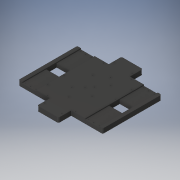
# Autodesk Inventor part: BottomPlateV2
Saved by Autodesk Inventor 2017 (Build 210142000, 142)
## iProperties
Created: 2017-03-10
Part Number: BottomPlateV2
Material: Polyethylene, High Density
Document SubType Name: Modeling
Designer: Naga
Density: 0.952 g/cm^3
Appearance: Smooth - Black
Author: Naga
Autodesk Inventor part; units mm, degrees
ref_plane "YZ Plane" through (0, 0, 0) normal (1, 0, 0) x (0, 1, 0)
ref_plane "XZ Plane" through (0, 0, 0) normal (0, 1, 0) x (-1, 0, 0)
ref_plane "XY Plane" through (0, 0, 0) normal (0, 0, 1) x (1, 0, 0)
sketch "Sketch1" plane through (0, 0, 0) normal (0, 1, 0) x (-1, 0, 0)
  line L0 (0, 0) -> (228.6, 0)
  line L1 (228.6, 0) -> (228.6, -228.6)
  line L2 (228.6, -228.6) -> (0, -228.6)
  line L3 (0, -228.6) -> (0, 0)
  line L4 (0, 0) -> (59.9999, 0)
  line L5 (59.9999, 0) -> (59.9999, -28.3972)
  line L6 (59.9999, -28.3972) -> (0, -28.3972)
  line L7 (0, -28.3972) -> (0, 0)
  line L8 (114.3, 0) -> (114.3, -114.3) construction
  line L9 (114.3, -114.3) -> (0, -114.3) construction
  line L10 (228.6, 0) -> (0, 0)
  line L11 (228.6, -228.6) -> (228.6, 0)
  line L12 (228.6, 0) -> (168.6001, 0)
  line L13 (168.6001, 0) -> (168.6001, -28.3972)
  line L14 (168.6001, -28.3972) -> (228.6, -28.3972)
  line L15 (228.6, -28.3972) -> (228.6, 0)
  line L16 (228.6, -228.6) -> (228.6, 0)
  line L17 (0, 0) -> (0, -228.6)
  line L18 (0, -228.6) -> (59.9999, -228.6)
  line L19 (59.9999, -228.6) -> (59.9999, -200.2028)
  line L20 (59.9999, -200.2028) -> (0, -200.2028)
  line L21 (0, -200.2028) -> (0, -228.6)
  line L22 (228.6, 0) -> (228.6, -228.6)
  line L23 (228.6, -228.6) -> (168.6001, -228.6)
  line L24 (168.6001, -228.6) -> (168.6001, -200.2028)
  line L25 (168.6001, -200.2028) -> (228.6, -200.2028)
  line L26 (228.6, -200.2028) -> (228.6, -228.6)
  dimension "d0" = 228.6
  dimension "d1" = 228.6
  dimension "d2" = 59.9999
  dimension "d3" = 28.3972
  constraints: 54 end point, 17 symmetric about line, 4 parallel, 2 horizontal, 2 midpoint, 2 perpendicular, 1 vertical
  measures "d0" distance of L1.end L2.end
  measures "d1" distance of L0.end L1.end
  measures "d2" distance of L5.end L6.end
  measures "d3" distance of L4.end L5.end
extrude "Extrusion1" add sketch "Sketch1" along normal blind 12.7 contours L0 L13 L14 L1 L25 L24 L2 L19 L20 L3 L6 L5
sketch "Sketch2" plane through (0, 12.7, 0) normal (0, 1, 0) x (1, 0, 0)
  line L0 (-59.9999, 200.2028) -> (-59.9999, 228.6) projected
  line L1 (-59.9999, 228.6) -> (-168.6001, 228.6) projected
  line L2 (-168.6001, 228.6) -> (-168.6001, 200.2028) projected
  line L3 (-168.6001, 200.2028) -> (-228.6, 200.2028) projected
  line L4 (-228.6, 200.2028) -> (-228.6, 28.3972) projected
  line L5 (-228.6, 28.3972) -> (-168.6001, 28.3972) projected
  line L6 (-168.6001, 28.3972) -> (-168.6001, 0) projected
  line L7 (-168.6001, 0) -> (-59.9999, 0) projected
  line L8 (-59.9999, 0) -> (-59.9999, 28.3972) projected
  line L9 (-59.9999, 28.3972) -> (0, 28.3972) projected
  line L10 (0, 28.3972) -> (0, 200.2028) projected
  line L11 (0, 200.2028) -> (-59.9999, 200.2028) projected
  line L12 (-228.6, 28.3972) -> (-168.6001, 28.3972) projected
  line L13 (-198.6001, 28.3972) -> (-198.6001, 34.7472) construction
  line L14 (-228.6, 200.2028) -> (-228.6, 28.3972) projected
  line L15 (-228.6, 34.7472) -> (-219.075, 34.7472) construction
  line L16 (-228.6, 34.7472) -> (-219.075, 34.7472) construction
  line L17 (-219.075, 34.7472) -> (-180.975, 34.7472)
  line L18 (-180.975, 34.7472) -> (-180.975, 44.2722)
  line L19 (-180.975, 44.2722) -> (-219.075, 44.2722)
  line L20 (-219.075, 44.2722) -> (-219.075, 34.7472)
  line L21 (-200.025, 44.2722) -> (-200.025, 39.5097) construction
  line L22 (-200.025, 39.5097) -> (-219.075, 39.5097) construction
  circle A0 centre (-200.025, 39.5097) radius 1.5875
  line L23 (-200.025, 39.5097) -> (-214.825, 39.5097)
  circle A1 centre (-214.825, 39.5097) radius 1.5875
  circle A2 centre (-185.225, 39.5097) radius 1.5875
  line L24 (-228.6, 200.2028) -> (-228.6, 28.3972) projected
  line L25 (-228.6, 114.3) -> (-114.3, 114.3) construction
  line L26 (-114.3, 114.3) -> (-114.3, 0) construction
  line L27 (-29.9999, 28.3972) -> (-29.9999, 34.7472) construction
  line L28 (0, 34.7472) -> (-9.525, 34.7472) construction
  line L29 (0, 34.7472) -> (-9.525, 34.7472) construction
  line L30 (-9.525, 34.7472) -> (-47.625, 34.7472)
  line L31 (-47.625, 34.7472) -> (-47.625, 44.2722)
  line L32 (-47.625, 44.2722) -> (-9.525, 44.2722)
  line L33 (-9.525, 44.2722) -> (-9.525, 34.7472)
  line L34 (-28.575, 44.2722) -> (-28.575, 39.5097) construction
  line L35 (-28.575, 39.5097) -> (-9.525, 39.5097) construction
  circle A3 centre (-28.575, 39.5097) radius 1.5875
  line L36 (-28.575, 39.5097) -> (-13.775, 39.5097)
  circle A4 centre (-13.775, 39.5097) radius 1.5875
  circle A5 centre (-43.375, 39.5097) radius 1.5875
  line L37 (-198.6001, 200.2028) -> (-198.6001, 193.8528) construction
  line L38 (-228.6, 193.8528) -> (-219.075, 193.8528) construction
  line L39 (-228.6, 193.8528) -> (-219.075, 193.8528) construction
  line L40 (-219.075, 193.8528) -> (-180.975, 193.8528)
  line L41 (-180.975, 193.8528) -> (-180.975, 184.3278)
  line L42 (-180.975, 184.3278) -> (-219.075, 184.3278)
  line L43 (-219.075, 184.3278) -> (-219.075, 193.8528)
  line L44 (-200.025, 184.3278) -> (-200.025, 189.0903) construction
  line L45 (-200.025, 189.0903) -> (-219.075, 189.0903) construction
  circle A6 centre (-200.025, 189.0903) radius 1.5875
  line L46 (-200.025, 189.0903) -> (-214.825, 189.0903)
  circle A7 centre (-214.825, 189.0903) radius 1.5875
  circle A8 centre (-185.225, 189.0903) radius 1.5875
  line L47 (-114.3, 114.3) -> (-114.3, 228.6) construction
  line L48 (-47.625, 193.8528) -> (-47.625, 184.3278)
  circle A9 centre (-43.375, 189.0903) radius 1.5875
  circle A10 centre (-28.575, 189.0903) radius 1.5875
  line L49 (-29.9999, 200.2028) -> (-29.9999, 193.8528) construction
  line L50 (-47.625, 184.3278) -> (-9.525, 184.3278)
  line L51 (-9.525, 184.3278) -> (-9.525, 193.8528)
  line L52 (0, 193.8528) -> (-9.525, 193.8528) construction
  line L53 (0, 193.8528) -> (-9.525, 193.8528) construction
  line L54 (-9.525, 193.8528) -> (-47.625, 193.8528)
  line L55 (-28.575, 189.0903) -> (-13.775, 189.0903)
  line L56 (-28.575, 189.0903) -> (-9.525, 189.0903) construction
  circle A11 centre (-13.775, 189.0903) radius 1.5875
  line L57 (-28.575, 184.3278) -> (-28.575, 189.0903) construction
  point P0 (0, 0)
  dimension "d6" = 6.35
  dimension "d7" = 9.525
  dimension "d8" = 0
  dimension "d9" = 38.1
  dimension "d10" = 9.525
  dimension "d11" = 3.175
  dimension "d12" = 14.8
  dimension "d13" = 3.175
  constraints: 86 end point, 47 symmetric about line, 12 centre point, 8 coincident, 5 midpoint, 5 point on line, 3 horizontal, 3 perpendicular, 2 parallel, 2 vertical, 1 collinear, 10 other
  measures "d6" distance of L13.start L13.end
  measures "d7" distance of L15.start L15.end
  measures "d8" distance between parallel lines of L15 L16
  measures "d9" distance of L19.end L18.end
  measures "d10" distance of L18.end L17.end
  measures "d11" diameter of A0
  measures "d12" distance of L23.start L23.end
  measures "d13" diameter of A1
extrude "Extrusion2" cut sketch "Sketch2" against normal blind 0.7937 contours L20 L19 L18 L17 | L30 L31 L32 L33 | L40 L41 L42 L43 | L54 L51 L50 L48
sketch "Sketch3" plane through (0, 0, 0) normal (0, -1, 0) x (1, 0, 0)
  circle A0 centre (-13.775, -39.5097) radius 1.5875 projected
  circle A1 centre (-28.575, -39.5097) radius 1.5875 projected
  circle A2 centre (-43.375, -39.5097) radius 1.5875 projected
  circle A3 centre (-13.775, -189.0903) radius 1.5875 projected
  circle A4 centre (-28.575, -189.0903) radius 1.5875 projected
  circle A5 centre (-43.375, -189.0903) radius 1.5875 projected
  circle A6 centre (-185.225, -189.0903) radius 1.5875 projected
  circle A7 centre (-200.025, -189.0903) radius 1.5875 projected
  circle A8 centre (-214.825, -189.0903) radius 1.5875 projected
  circle A9 centre (-214.825, -39.5097) radius 1.5875 projected
  circle A10 centre (-200.025, -39.5097) radius 1.5875 projected
  circle A11 centre (-185.225, -39.5097) radius 1.5875 projected
  point P0 (0, 0)
extrude "Extrusion3" cut sketch "Sketch3" against normal up to surface (12.7 mm away)
sketch "Sketch4" plane through (0, 12.7, 0) normal (0, 1, 0) x (1, 0, 0)
  line L0 (-219.075, 184.3278) -> (-219.075, 193.8528) projected
  line L1 (-219.075, 193.8528) -> (-180.975, 193.8528)
  line L2 (-180.975, 193.8528) -> (-180.975, 34.7472)
  line L3 (-180.975, 34.7472) -> (-219.075, 34.7472)
  line L4 (-219.075, 34.7472) -> (-219.075, 193.8528)
  line L5 (-47.625, 193.8528) -> (-9.525, 193.8528) projected
  line L6 (-9.525, 44.2722) -> (-9.525, 34.7472) projected
  line L7 (-47.625, 193.8528) -> (-9.525, 193.8528)
  line L8 (-9.525, 193.8528) -> (-9.525, 34.7472)
  line L9 (-9.525, 34.7472) -> (-47.625, 34.7472)
  line L10 (-47.625, 34.7472) -> (-47.625, 193.8528)
  point P0 (0, 0)
  constraints: 16 end point, 4 parallel, 2 horizontal, 2 perpendicular
extrude "Extrusion4" cut sketch "Sketch4" against normal blind 3.175
sketch "Sketch5" plane through (0, 12.7, 0) normal (0, 1, 0) x (1, 0, 0)
  line L0 (-168.6001, 0) -> (-59.9999, 0) projected
  line L1 (-114.3, 0) -> (-114.3, 38.1)
  line L2 (-228.6, 200.2028) -> (-228.6, 28.3972) projected
  line L3 (-228.6, 38.1) -> (-152.4, 38.1)
  circle A0 centre (-152.4, 38.1) radius 1.5875
  line L4 (-228.6, 114.3) -> (-127.0378, 114.3)
  circle A1 centre (-76.2, 38.1) radius 1.5875
  circle A2 centre (-152.4, 190.5) radius 1.5875
  circle A3 centre (-76.2, 190.5) radius 1.5875
  point P0 (0, 0)
  dimension "d20" = 38.1
  dimension "d21" = 76.2
  dimension "d22" = 3.175
  constraints: 6 end point, 4 centre point, 4 symmetric about line, 2 coincident, 2 horizontal, 2 midpoint, 1 parallel, 1 point on line, 3 other
  measures "d20" distance of L1.start L1.end
  measures "d21" distance of L3.start L3.end
  measures "d22" diameter of A0
extrude "Extrusion5" cut sketch "Sketch5" against normal up to surface (12.7 mm away)
sketch "Sketch7" plane through (0, 12.7, 0) normal (0, 1, 0) x (1, 0, 0)
  circle A0 centre (-152.4, 190.5) radius 1.5875 projected
  circle A1 centre (-76.2, 190.5) radius 1.5875 projected
  circle A2 centre (-76.2, 38.1) radius 1.5875 projected
  circle A3 centre (-152.4, 38.1) radius 1.5875 projected
  line L0 (-59.9999, 200.2028) -> (-59.9999, 228.6) projected
  line L1 (-59.9999, 228.6) -> (-168.6001, 228.6) projected
  line L2 (-168.6001, 228.6) -> (-168.6001, 200.2028) projected
  line L3 (-168.6001, 200.2028) -> (-228.6, 200.2028) projected
  line L4 (-228.6, 200.2028) -> (-228.6, 28.3972) projected
  line L5 (-228.6, 28.3972) -> (-168.6001, 28.3972) projected
  line L6 (-168.6001, 28.3972) -> (-168.6001, 0) projected
  line L7 (-168.6001, 0) -> (-59.9999, 0) projected
  line L8 (-59.9999, 0) -> (-59.9999, 28.3972) projected
  line L9 (-59.9999, 28.3972) -> (0, 28.3972) projected
  line L10 (0, 28.3972) -> (0, 200.2028) projected
  line L11 (0, 200.2028) -> (-59.9999, 200.2028) projected
  line L12 (-47.625, 34.7472) -> (-47.625, 193.8528) projected
  line L13 (-47.625, 193.8528) -> (-9.525, 193.8528) projected
  line L14 (-9.525, 193.8528) -> (-9.525, 34.7472) projected
  line L15 (-9.525, 34.7472) -> (-47.625, 34.7472) projected
  line L16 (-219.075, 34.7472) -> (-219.075, 193.8528) projected
  line L17 (-219.075, 193.8528) -> (-180.975, 193.8528) projected
  line L18 (-180.975, 193.8528) -> (-180.975, 34.7472) projected
  line L19 (-180.975, 34.7472) -> (-219.075, 34.7472) projected
  line L20 (-228.6, 228.6) -> (-142.875, 228.6)
  line L21 (-228.6, 200.2028) -> (-228.6, 228.6)
  line L22 (0, 228.6) -> (-85.725, 228.6)
  line L23 (0, 200.2028) -> (0, 228.6)
  line L24 (0, 0) -> (-85.725, 0)
  line L25 (-85.725, 0) -> (-85.725, 34.7472)
  line L26 (-85.725, 34.7472) -> (0, 34.7472)
  line L27 (0, 34.7472) -> (0, 0)
  line L28 (-228.6, 0) -> (-142.875, 0)
  line L29 (-142.875, 0) -> (-142.875, 34.7472)
  line L30 (-142.875, 34.7472) -> (-228.6, 34.7472)
  line L31 (-228.6, 34.7472) -> (-228.6, 0)
  line L32 (-228.6, 228.6) -> (-142.875, 228.6)
  line L33 (-142.875, 228.6) -> (-142.875, 193.8528)
  line L34 (-142.875, 193.8528) -> (-228.6, 193.8528)
  line L35 (-228.6, 193.8528) -> (-228.6, 228.6)
  line L36 (0, 28.3972) -> (0, 200.2028) projected
  line L37 (0, 193.8528) -> (-85.725, 193.8528)
  line L38 (-85.725, 193.8528) -> (-85.725, 228.6)
  line L39 (-85.725, 228.6) -> (0, 228.6)
  line L40 (0, 228.6) -> (0, 193.8528)
  dimension "d30" = 34.7472
  constraints: 40 end point, 8 parallel, 6 horizontal, 4 perpendicular, 4 point on line
  measures "d30" distance of L24.end L25.end
extrude "Extrusion7" cut sketch "Sketch7" against normal blind 25.4 contours L11 L10 L37 L13 L38 L1 L0 | L0 L22 L23 L11 | L33 L34 L17 L4 L3 L2 L1 | L10 L9 L8 L7 L25 L26 L15 | L2 L3 L21 L20 | L27 L24 L8 L9 | L30 L29 L7 L6 L5 L4 L19 | L5 L6 L28 L31
sketch "Sketch8" plane through (0, 12.7, 0) normal (0, 1, 0) x (1, 0, 0)
  circle A0 centre (-214.825, 189.0903) radius 1.5875 projected
  circle A1 centre (-185.225, 189.0903) radius 1.5875 projected
  circle A2 centre (-28.575, 189.0903) radius 1.5875 projected
  circle A3 centre (-43.375, 39.5097) radius 1.5875 projected
  circle A4 centre (-13.775, 39.5097) radius 1.5875 projected
  circle A5 centre (-28.575, 39.5097) radius 1.5875 projected
  circle A6 centre (-13.775, 189.0903) radius 1.5875 projected
  circle A7 centre (-43.375, 189.0903) radius 1.5875 projected
  circle A8 centre (-200.025, 189.0903) radius 1.5875 projected
  circle A9 centre (-214.825, 39.5097) radius 1.5875 projected
  circle A10 centre (-185.225, 39.5097) radius 1.5875 projected
  circle A11 centre (-200.025, 39.5097) radius 1.5875 projected
  circle A12 centre (-152.4, 38.1) radius 1.5875 projected
  circle A13 centre (-76.2, 38.1) radius 1.5875 projected
  circle A14 centre (-76.2, 190.5) radius 1.5875 projected
  circle A15 centre (-152.4, 190.5) radius 1.5875 projected
  line L0 (-142.875, 0) -> (-142.875, 34.7472) projected
  line L1 (-142.875, 34.7472) -> (-228.6, 34.7472) projected
  line L2 (-228.6, 193.8528) -> (-228.6, 34.7472) projected
  line L3 (-228.6, 193.8528) -> (-142.875, 193.8528) projected
  line L4 (-142.875, 193.8528) -> (-142.875, 228.6) projected
  line L5 (-85.725, 228.6) -> (-142.875, 228.6) projected
  line L6 (-85.725, 228.6) -> (-85.725, 193.8528) projected
  line L7 (-85.725, 193.8528) -> (0, 193.8528) projected
  line L8 (0, 34.7472) -> (0, 193.8528) projected
  line L9 (0, 34.7472) -> (-85.725, 34.7472) projected
  line L10 (-85.725, 34.7472) -> (-85.725, 0) projected
  line L11 (-142.875, 0) -> (-85.725, 0) projected
  line L12 (-142.875, 0) -> (-85.725, 0) projected
  line L13 (-142.875, 0) -> (-138.5062, 0)
  line L14 (-138.5062, 0) -> (-138.5062, 89.9922)
  line L15 (-138.5062, 89.9922) -> (-142.875, 89.9922)
  line L16 (-142.875, 89.9922) -> (-142.875, 0)
  line L17 (-142.875, 0) -> (-142.875, 34.7472) projected
  line L18 (-138.5062, 0) -> (-142.875, 0)
  line L19 (-142.875, 0) -> (-142.875, 16.002)
  line L20 (-142.875, 16.002) -> (-138.5062, 16.002)
  line L21 (-138.5062, 16.002) -> (-138.5062, 0)
  line L22 (-85.725, 0) -> (-90.0938, 0)
  line L23 (-90.0938, 0) -> (-90.0938, 14.5034)
  line L24 (-90.0938, 14.5034) -> (-85.725, 14.5034)
  line L25 (-85.725, 14.5034) -> (-85.725, 0)
  line L26 (-85.725, 0) -> (-90.0938, 0)
  line L27 (-90.0938, 0) -> (-90.0938, 96.4946)
  line L28 (-90.0938, 96.4946) -> (-85.725, 96.4946)
  line L29 (-85.725, 96.4946) -> (-85.725, 0)
  circle A16 centre (-138.5062, 89.9922) radius 1.5875
  circle A17 centre (-90.0938, 96.4946) radius 1.5875
  circle A18 centre (-90.0938, 14.5034) radius 1.5875
  circle A19 centre (-138.5062, 16.002) radius 1.5875
  point P0 (0, 0)
  dimension "d33" = 4.3688
  dimension "d34" = 89.9922
  dimension "d35" = 16.002
  dimension "d36" = 4.3688
  dimension "d37" = 14.5034
  dimension "d38" = 96.4946
  dimension "d39" = 3.175
  dimension "d40" = 3.175
  dimension "d41" = 3.175
  dimension "d42" = 3.175
  dimension "d74" = 4.3688
  constraints: 32 end point, 8 parallel, 4 centre point, 4 coincident, 4 horizontal, 4 perpendicular, 1 point on line
  measures "d33" distance of L15.end L14.end
  measures "d34" distance of L14.end L13.end
  measures "d35" distance of L18.end L19.end
  measures "d36" distance of L23.end L24.end
  measures "d37" distance of L22.end L23.end
  measures "d38" distance of L26.end L27.end
  measures "d39" diameter of A16
  measures "d40" diameter of A17
  measures "d41" diameter of A18
  measures "d42" diameter of A19
  measures "d74" distance of L27.end L28.end
extrude "ardMount" cut sketch "Sketch8" against normal up to surface (12.7 mm away) contours A19 L14 L20 | L20 L14 A19 | L14 A19 | A18 L27 L23 | L23 L24 A18 | A16 L14 L15 | L15 L14 A16 | L27 A18 L24 | A17 L28 L27 | L27 L28 A17
sketch "Sketch9" plane through (0, 12.7, 0) normal (0, 1, 0) x (1, 0, 0)
  circle A0 centre (-138.5062, 16.002) radius 1.5875 projected
  circle A1 centre (-90.0938, 14.5034) radius 1.5875 projected
  circle A2 centre (-138.5062, 89.9922) radius 1.5875 projected
  circle A3 centre (-90.0938, 96.4946) radius 1.5875 projected
  line L0 (-142.875, 34.7472) -> (-142.875, 0) projected
  line L1 (-142.875, 0) -> (-85.725, 0) projected
  line L2 (-85.725, 0) -> (-85.725, 34.7472) projected
  line L3 (-85.725, 34.7472) -> (-47.625, 34.7472) projected
  line L4 (-47.625, 34.7472) -> (-47.625, 193.8528) projected
  line L5 (-47.625, 193.8528) -> (-85.725, 193.8528) projected
  line L6 (-85.725, 193.8528) -> (-85.725, 228.6) projected
  line L7 (-85.725, 228.6) -> (-142.875, 228.6) projected
  line L8 (-142.875, 228.6) -> (-142.875, 193.8528) projected
  line L9 (-142.875, 193.8528) -> (-180.975, 193.8528) projected
  line L10 (-180.975, 193.8528) -> (-180.975, 34.7472) projected
  line L11 (-180.975, 34.7472) -> (-142.875, 34.7472) projected
  circle A4 centre (-152.4, 190.5) radius 1.5875 projected
  circle A5 centre (-76.2, 190.5) radius 1.5875 projected
  circle A6 centre (-76.2, 38.1) radius 1.5875 projected
  circle A7 centre (-152.4, 38.1) radius 1.5875 projected
  line L12 (-85.725, 228.6) -> (-142.875, 228.6) projected
  line L13 (-114.3, 228.6) -> (-114.3, 148.6607) construction
  line L14 (-142.875, 228.6) -> (-138.7856, 228.6) construction
  line L15 (-138.7856, 228.6) -> (-138.7856, 204.978) construction
  line L16 (-138.7856, 204.978) -> (-142.875, 204.978) construction
  line L17 (-142.875, 204.978) -> (-142.875, 228.6) construction
  line L18 (-142.875, 228.6) -> (-142.875, 193.8528) construction
  line L19 (-142.875, 228.6) -> (-138.7856, 228.6) construction
  line L20 (-138.7856, 228.6) -> (-138.7856, 147.066) construction
  line L21 (-138.7856, 147.066) -> (-142.875, 147.066) construction
  line L22 (-142.875, 147.066) -> (-142.875, 228.6) construction
  circle A8 centre (-138.7856, 204.978) radius 1.5875
  circle A9 centre (-138.7856, 147.066) radius 1.5875
  circle A10 centre (-89.8144, 204.978) radius 1.5875
  circle A11 centre (-89.8144, 147.066) radius 1.5875
  point P0 (0, 0)
  dimension "d45" = 4.0894
  dimension "d46" = 23.622
  dimension "d47" = 81.534
  dimension "d48" = 3.175
  dimension "d49" = 3.175
  constraints: 18 end point, 4 centre point, 4 parallel, 2 coincident, 2 horizontal, 2 perpendicular, 2 symmetric about line, 1 midpoint, 1 point on line, 1 vertical, 2 other
  measures "d45" distance of L15.end L16.end
  measures "d46" distance of L14.end L15.end
  measures "d47" distance of L19.end L20.end
  measures "d48" diameter of A8
  measures "d49" diameter of A9
extrude "piMount" cut sketch "Sketch9" against normal up to surface (12.7 mm away) contours A8 | A9 | A10 | A11
sketch "Sketch10" plane through (0, 0, 0) normal (0, -1, 0) x (1, 0, 0)
  circle A0 centre (-89.8144, -204.978) radius 1.5875 projected
  circle A1 centre (-89.8144, -147.066) radius 1.5875 projected
  circle A2 centre (-138.7856, -147.066) radius 1.5875 projected
  circle A3 centre (-138.7856, -204.978) radius 1.5875 projected
  circle A4 centre (-138.5062, -16.002) radius 1.5875 projected
  circle A5 centre (-90.0938, -14.5034) radius 1.5875 projected
  circle A6 centre (-138.5062, -89.9922) radius 1.5875 projected
  circle A7 centre (-90.0938, -96.4946) radius 1.5875 projected
  circle A8 centre (-214.825, -189.0903) radius 1.5875 projected
  circle A9 centre (-185.225, -189.0903) radius 1.5875 projected
  circle A10 centre (-28.575, -189.0903) radius 1.5875 projected
  circle A11 centre (-43.375, -39.5097) radius 1.5875 projected
  circle A12 centre (-13.775, -39.5097) radius 1.5875 projected
  circle A13 centre (-28.575, -39.5097) radius 1.5875 projected
  circle A14 centre (-13.775, -189.0903) radius 1.5875 projected
  circle A15 centre (-43.375, -189.0903) radius 1.5875 projected
  circle A16 centre (-200.025, -189.0903) radius 1.5875 projected
  circle A17 centre (-214.825, -39.5097) radius 1.5875 projected
  circle A18 centre (-185.225, -39.5097) radius 1.5875 projected
  circle A19 centre (-200.025, -39.5097) radius 1.5875 projected
  circle A20 centre (-152.4, -38.1) radius 1.5875 projected
  circle A21 centre (-76.2, -38.1) radius 1.5875 projected
  circle A22 centre (-76.2, -190.5) radius 1.5875 projected
  circle A23 centre (-152.4, -190.5) radius 1.5875 projected
  line L0 (-142.875, 0) -> (-142.875, -34.7472) projected
  line L1 (-142.875, -34.7472) -> (-228.6, -34.7472) projected
  line L2 (-228.6, -193.8528) -> (-228.6, -34.7472) projected
  line L3 (-228.6, -193.8528) -> (-142.875, -193.8528) projected
  line L4 (-142.875, -193.8528) -> (-142.875, -228.6) projected
  line L5 (-85.725, -228.6) -> (-142.875, -228.6) projected
  line L6 (-85.725, -228.6) -> (-85.725, -193.8528) projected
  line L7 (-85.725, -193.8528) -> (0, -193.8528) projected
  line L8 (0, -34.7472) -> (0, -193.8528) projected
  line L9 (0, -34.7472) -> (-85.725, -34.7472) projected
  line L10 (-85.725, -34.7472) -> (-85.725, 0) projected
  line L11 (-142.875, 0) -> (-85.725, 0) projected
  line L12 (-142.875, -34.7472) -> (-228.6, -34.7472) construction
  line L13 (-228.6, -34.7472) -> (-177.1396, -34.7472) construction
  line L14 (-177.1396, -34.7472) -> (-177.1396, -107.3912) construction
  line L15 (-177.1396, -107.3912) -> (-228.6, -107.3912) construction
  line L16 (-228.6, -107.3912) -> (-228.6, -34.7472) construction
  line L17 (-228.6, -34.7472) -> (-177.1396, -34.7472) construction
  line L18 (-177.1396, -34.7472) -> (-177.1396, -63.1952) construction
  line L19 (-177.1396, -63.1952) -> (-228.6, -63.1952) construction
  line L20 (-228.6, -63.1952) -> (-228.6, -34.7472) construction
  line L21 (-228.6, -34.7472) -> (-120.015, -34.7472) construction
  line L22 (-120.015, -34.7472) -> (-120.015, -107.3912) construction
  line L23 (-120.015, -107.3912) -> (-228.6, -107.3912) construction
  line L24 (-228.6, -107.3912) -> (-228.6, -34.7472) construction
  line L25 (-228.6, -34.7472) -> (-120.015, -34.7472) construction
  line L26 (-120.015, -34.7472) -> (-120.015, -63.1952) construction
  line L27 (-120.015, -63.1952) -> (-228.6, -63.1952) construction
  line L28 (-228.6, -63.1952) -> (-228.6, -34.7472) construction
  line L29 (-85.725, -193.8528) -> (0, -193.8528) construction
  line L30 (0, -193.8528) -> (-51.4604, -193.8528) construction
  line L31 (-51.4604, -193.8528) -> (-51.4604, -121.2088) construction
  line L32 (-51.4604, -121.2088) -> (0, -121.2088) construction
  line L33 (0, -121.2088) -> (0, -193.8528) construction
  line L34 (0, -34.7472) -> (0, -193.8528) construction
  line L35 (0, -193.8528) -> (-51.4604, -193.8528) construction
  line L36 (-51.4604, -193.8528) -> (-51.4604, -165.4048) construction
  line L37 (-51.4604, -165.4048) -> (0, -165.4048) construction
  line L38 (0, -165.4048) -> (0, -193.8528) construction
  line L39 (0, -193.8528) -> (-108.585, -193.8528) construction
  line L40 (-108.585, -193.8528) -> (-108.585, -121.2342) construction
  line L41 (-108.585, -121.2342) -> (0, -121.2342) construction
  line L42 (0, -121.2342) -> (0, -193.8528) construction
  line L43 (0, -193.8528) -> (-108.585, -193.8528) construction
  line L44 (-108.585, -193.8528) -> (-108.585, -165.4048) construction
  line L45 (-108.585, -165.4048) -> (0, -165.4048) construction
  line L46 (0, -165.4048) -> (0, -193.8528) construction
  circle A24 centre (-108.585, -121.2342) radius 1.5875
  circle A25 centre (-108.585, -165.4048) radius 1.5875
  circle A26 centre (-51.4604, -165.4048) radius 1.5875
  circle A27 centre (-51.4604, -121.2088) radius 1.5875
  circle A28 centre (-177.1396, -107.3912) radius 1.5875
  circle A29 centre (-177.1396, -63.1952) radius 1.5875
  circle A30 centre (-120.015, -63.1952) radius 1.5875
  circle A31 centre (-120.015, -107.3912) radius 1.5875
  point P0 (0, 0)
  dimension "d52" = 51.4604
  dimension "d53" = 72.644
  dimension "d54" = 28.448
  dimension "d55" = 108.585
  dimension "d56" = 51.4604
  dimension "d57" = 72.644
  dimension "d58" = 28.448
  dimension "d59" = 108.585
  dimension "d60" = 3.175
  dimension "d61" = 3.175
  dimension "d62" = 3.175
  dimension "d63" = 3.175
  dimension "d64" = 3.175
  dimension "d65" = 3.175
  dimension "d66" = 3.175
  dimension "d67" = 3.175
  constraints: 64 end point, 16 parallel, 8 centre point, 8 coincident, 8 horizontal, 8 perpendicular, 7 point on line
  measures "d52" distance of L14.end L15.end
  measures "d53" distance of L13.end L14.end
  measures "d54" distance of L17.end L18.end
  measures "d55" distance of L22.end L23.end
  measures "d56" distance of L31.end L32.end
  measures "d57" distance of L30.end L31.end
  measures "d58" distance of L35.end L36.end
  measures "d59" distance of L40.end L41.end
  measures "d60" diameter of A24
  measures "d61" diameter of A25
  measures "d62" diameter of A26
  measures "d63" diameter of A27
  measures "d64" diameter of A28
  measures "d65" diameter of A29
  measures "d66" diameter of A30
  measures "d67" diameter of A31
extrude "sabertoothMount" cut sketch "Sketch10" against normal up to surface (12.7 mm away) contours A24 | A25 | A26 | A27 | A28 | A29 | A30 | A31
sketch "Sketch11" plane through (0, 0, 0) normal (0, -1, 0) x (1, 0, 0)
  line L0 (-47.625, -34.7472) -> (-47.625, -193.8528) projected
  circle A0 centre (-120.015, -63.1952) radius 1.5875 projected
  circle A1 centre (-120.015, -107.3912) radius 1.5875 projected
  circle A2 centre (-177.1396, -63.1952) radius 1.5875 projected
  circle A3 centre (-51.4604, -121.2088) radius 1.5875 projected
  circle A4 centre (-108.585, -165.4048) radius 1.5875 projected
  circle A5 centre (-108.585, -121.2342) radius 1.5875 projected
  circle A6 centre (-51.4604, -165.4048) radius 1.5875 projected
  circle A7 centre (-177.1396, -107.3912) radius 1.5875 projected
  circle A8 centre (-89.8144, -204.978) radius 1.5875 projected
  circle A9 centre (-89.8144, -147.066) radius 1.5875 projected
  circle A10 centre (-138.7856, -147.066) radius 1.5875 projected
  circle A11 centre (-138.7856, -204.978) radius 1.5875 projected
  circle A12 centre (-138.5062, -16.002) radius 1.5875 projected
  circle A13 centre (-90.0938, -14.5034) radius 1.5875 projected
  circle A14 centre (-138.5062, -89.9922) radius 1.5875 projected
  circle A15 centre (-90.0938, -96.4946) radius 1.5875 projected
  circle A16 centre (-214.825, -189.0903) radius 1.5875 projected
  circle A17 centre (-185.225, -189.0903) radius 1.5875 projected
  circle A18 centre (-28.575, -189.0903) radius 1.5875 projected
  circle A19 centre (-43.375, -39.5097) radius 1.5875 projected
  circle A20 centre (-13.775, -39.5097) radius 1.5875 projected
  circle A21 centre (-28.575, -39.5097) radius 1.5875 projected
  circle A22 centre (-13.775, -189.0903) radius 1.5875 projected
  circle A23 centre (-43.375, -189.0903) radius 1.5875 projected
  circle A24 centre (-200.025, -189.0903) radius 1.5875 projected
  circle A25 centre (-214.825, -39.5097) radius 1.5875 projected
  circle A26 centre (-185.225, -39.5097) radius 1.5875 projected
  circle A27 centre (-200.025, -39.5097) radius 1.5875 projected
  circle A28 centre (-152.4, -38.1) radius 1.5875 projected
  circle A29 centre (-76.2, -38.1) radius 1.5875 projected
  circle A30 centre (-76.2, -190.5) radius 1.5875 projected
  circle A31 centre (-152.4, -190.5) radius 1.5875 projected
  line L1 (-142.875, 0) -> (-142.875, -34.7472) projected
  line L2 (-142.875, -34.7472) -> (-228.6, -34.7472) projected
  line L3 (-228.6, -193.8528) -> (-228.6, -34.7472) projected
  line L4 (-228.6, -193.8528) -> (-142.875, -193.8528) projected
  line L5 (-142.875, -193.8528) -> (-142.875, -228.6) projected
  line L6 (-85.725, -228.6) -> (-142.875, -228.6) projected
  line L7 (-85.725, -228.6) -> (-85.725, -193.8528) projected
  line L8 (-85.725, -193.8528) -> (0, -193.8528) projected
  line L9 (0, -34.7472) -> (0, -193.8528) projected
  line L10 (0, -34.7472) -> (-85.725, -34.7472) projected
  line L11 (-85.725, -34.7472) -> (-85.725, 0) projected
  line L12 (-142.875, 0) -> (-85.725, 0) projected
  line L13 (-180.975, -193.8528) -> (-180.975, -34.7472) projected
  line L14 (-219.075, -34.7472) -> (-219.075, -193.8528) projected
  line L15 (-9.525, -193.8528) -> (-9.525, -34.7472) projected
  line L16 (0, -34.7472) -> (0, -193.8528) construction
  line L17 (0, -114.3) -> (-228.6, -114.3) construction
  line L18 (-228.6, -193.8528) -> (-228.6, -34.7472) construction
  line L19 (-47.625, -34.7472) -> (-47.625, -193.8528) construction
  line L20 (-47.625, -114.3) -> (-9.525, -114.3) construction
  line L21 (-9.525, -100.0125) -> (-47.625, -100.0125)
  line L22 (-47.625, -100.0125) -> (-47.625, -128.5875)
  line L23 (-47.625, -128.5875) -> (-9.525, -128.5875)
  line L24 (-9.525, -128.5875) -> (-9.525, -100.0125)
  line L25 (-9.525, -100.0125) -> (-47.625, -128.5875) construction
  line L26 (-47.625, -100.0125) -> (-9.525, -128.5875) construction
  line L27 (-180.9463, -100.0125) -> (-219.075, -100.0125)
  line L28 (-219.075, -100.0125) -> (-219.075, -128.5875)
  line L29 (-219.075, -128.5875) -> (-180.9463, -128.5875)
  line L30 (-180.9463, -128.5875) -> (-180.9463, -100.0125)
  line L31 (-180.9463, -100.0125) -> (-219.075, -128.5875) construction
  line L32 (-219.075, -100.0125) -> (-180.9463, -128.5875) construction
  point P0 (0, 0)
  point P1 (-28.575, -114.3)
  point P2 (-200.0106, -114.3)
  dimension "d70" = 28.575
  constraints: 28 end point, 9 midpoint, 5 point on line, 4 parallel, 2 horizontal, 2 perpendicular
  measures "d70" distance of L22.end L21.end
extrude "Extrusion11" cut sketch "Sketch11" against normal up to surface (9.525 mm away) contours L21 L15 L23 L0 | L27 L30 L29 L13 | L13 L29 L14 L27
fillet "Fillet1" radius 3.175 8 edges at (-142.875, 6.35, 0) (-85.725, 6.35, 0) (-85.725, 6.35, -228.6) (0, 6.35, -34.7472) (0, 6.35, -193.8528) (-142.875, 6.35, -228.6) (-228.6, 6.35, -193.8528) (-228.6, 6.35, -34.7472)
body "Solid1"
